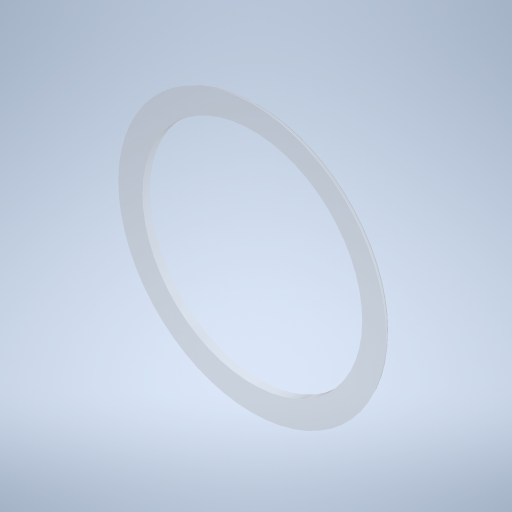
# Autodesk Inventor part: riduttore
Saved by Autodesk Inventor 2023 (Build 270158000, 158)
## iProperties
Created: 2023-08-19
Part Number: riduttore
Material: Plastica PET
Document SubType Name: Modeling
Designer: Admin
Density: 1.541 g/cm^3
Appearance: Policarbonato - Trasparente
Author: Admin
Autodesk Inventor part; units mm, degrees
ref_plane "YZ Plane" through (0, 0, 0) normal (1, 0, 0) x (0, 1, 0)
ref_plane "XZ Plane" through (0, 0, 0) normal (0, 1, 0) x (-1, 0, 0)
ref_plane "XY Plane" through (0, 0, 0) normal (0, 0, 1) x (1, 0, 0)
sketch "Schizzo1" plane through (0, 0, 0) normal (0, 0, 1) x (1, 0, 0)
  arc A0 (-10.1491, -19.2369) -> (-10.8943, -18.8249) centre (0, 0) ccw construction
  circle A1 centre (-4.8008, -2.5783) radius 24.7387 projected
  circle A2 centre (-4.8008, -2.5783) radius 21.75
  circle A3 centre (-4.8008, -2.5783) radius 24.7387
  circle A4 centre (0, 0) radius 20.5283 construction
  circle A5 centre (-4.8223, -2.7567) radius 25.8195 projected
  circle A6 centre (-4.8223, -2.7567) radius 25.8195
  circle A7 centre (-4.8223, -2.7567) radius 26.5
  point P0 (0, 0)
  point P1 (7.8094, -20.2997)
  point P2 (-12.6102, 17.7213)
  point P3 (9.3339, 19.6454)
  point P4 (21.6646, -1.9253)
  point P5 (20.6959, -6.6889)
  point P6 (4.7376, 21.2278)
  dimension "d4" = 53
  constraints: 4 centre point, 4 coincident, 3 equal radius
  measures "d4" diameter of A7
extrude "Estrusione1" add sketch "Schizzo1" against normal blind 1.5 contours A1 | A5 | A7
fillet "Raccordo1" radius 2 1 edges at (-31.3223, -2.7567, -1.5)
